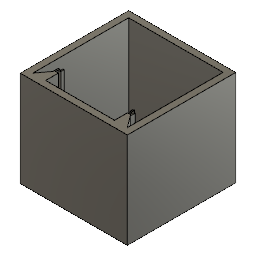
Albapod-V1 (Autodesk Fusion 360 design; units mm, degrees)
Autodesk Fusion 360 part; units mm, degrees
sketch "Sketch1" plane through (0, 0, 0) normal (0, 1, 0) x (1, 0, 0)
  line L0 (0, 0) -> (1, 0)
  line L1 (1, 0) -> (1, -1.5)
  line L2 (1, -1.5) -> (0, -1.5)
  line L3 (0, -1.5) -> (0, 0)
  line L4 (1, -1.5) -> (-2.25, -1.5)
  line L5 (-2.25, -1.5) -> (-2.25, -2.5)
  line L6 (-2.25, -2.5) -> (1, -2.5)
  line L7 (1, -2.5) -> (1, -1.5)
  line L8 (-2.25, -2.5) -> (-1.25, -2.5)
  line L9 (-1.25, -2.5) -> (-1.25, -4.5)
  line L10 (-1.25, -4.5) -> (-2.25, -4.5)
  line L11 (-2.25, -4.5) -> (-2.25, -2.5)
  line L12 (-2.25, -4.5) -> (1, -4.5)
  line L13 (1, -4.5) -> (1, -5.5)
  line L14 (1, -5.5) -> (-2.25, -5.5)
  line L15 (-2.25, -5.5) -> (-2.25, -4.5)
  line L16 (1, -5.5) -> (0, -5.5)
  line L17 (0, -5.5) -> (0, -14.5)
  line L18 (0, -14.5) -> (1, -14.5)
  line L19 (1, -14.5) -> (1, -5.5)
  line L20 (55, 0) -> (56, 0)
  line L21 (56, 0) -> (56, -1.5)
  line L22 (56, -1.5) -> (55, -1.5)
  line L23 (55, -1.5) -> (55, 0)
  line L24 (55, -1.5) -> (58.25, -1.5)
  line L25 (58.25, -1.5) -> (58.25, -2.5)
  line L26 (58.25, -2.5) -> (55, -2.5)
  line L27 (55, -2.5) -> (55, -1.5)
  line L28 (58.25, -2.5) -> (57.25, -2.5)
  line L29 (57.25, -2.5) -> (57.25, -4.5)
  line L30 (57.25, -4.5) -> (58.25, -4.5)
  line L31 (58.25, -4.5) -> (58.25, -2.5)
  line L32 (58.25, -4.5) -> (55, -4.5)
  line L33 (55, -4.5) -> (55, -5.5)
  line L34 (55, -5.5) -> (58.25, -5.5)
  line L35 (58.25, -5.5) -> (58.25, -4.5)
  line L36 (55, -5.5) -> (56, -5.5)
  line L37 (56, -5.5) -> (56, -14.5)
  line L38 (56, -14.5) -> (55, -14.5)
  line L39 (55, -14.5) -> (55, -5.5)
  line L40 (-9, -14.5) -> (65, -14.5)
  line L41 (65, -14.5) -> (65, 60.5)
  line L42 (65, 60.5) -> (-9, 60.5)
  line L43 (-9, 60.5) -> (-9, -14.5)
  line L44 (70, -19.5) -> (70, 65.5)
  line L45 (70, 65.5) -> (-14, 65.5)
  line L46 (-14, 65.5) -> (-14, -19.5)
  line L47 (-14, -19.5) -> (70, -19.5)
  line L48 (-2.25, -5.5) -> (-9, -14.5)
  line L49 (58.25, -5.5) -> (65, -14.5)
  dimension "d1" = 1
  dimension "d2" = 1.5
  dimension "d3" = 3.25
  dimension "d4" = 1
  dimension "d5" = 1
  dimension "d6" = 2
  dimension "d7" = 3.25
  dimension "d8" = 1
  dimension "d9" = 9
  dimension "d10" = 1.5
  dimension "d11" = 54
  dimension "d12" = 3.25
  dimension "d13" = 1
  dimension "d14" = 2
  dimension "d15" = 3.25
  dimension "d16" = 1
  dimension "d17" = 9
  dimension "d18" = 74
  dimension "d19" = 75
  dimension "d20" = 10
  dimension "d21" = 60.5
  dimension "d22" = 5
  constraint horizontal L0
  constraint vertical L1
  constraint horizontal L2
  constraint vertical L3
  constraint coincident L0.start L3.end
  constraint horizontal L4
  constraint vertical L5
  constraint horizontal L6
  constraint vertical L7
  constraint horizontal L8
  constraint vertical L9
  constraint horizontal L10
  constraint vertical L11
  constraint horizontal L12
  constraint vertical L13
  constraint horizontal L14
  constraint vertical L15
  constraint horizontal L16
  constraint vertical L17
  constraint horizontal L18
  constraint vertical L19
  constraint horizontal L20
  constraint vertical L21
  constraint horizontal L22
  constraint vertical L23
  constraint horizontal L24
  constraint vertical L25
  constraint horizontal L26
  constraint vertical L27
  constraint horizontal L28
  constraint vertical L29
  constraint horizontal L30
  constraint vertical L31
  constraint horizontal L32
  constraint vertical L33
  constraint horizontal L34
  constraint vertical L35
  constraint horizontal L36
  constraint vertical L37
  constraint horizontal L38
  constraint vertical L39
  constraint horizontal L40
  constraint vertical L41
  constraint horizontal L42
  constraint vertical L43
  measures "d1" distance of L0.start L0.end
  measures "d2" distance of L0.start L2.end
  measures "d3" distance of L1.end L4.end
  measures "d4" distance of L1.end L6.end
  measures "d5" distance of L5.end L8.end
  measures "d6" distance of L5.end L10.end
  measures "d7" distance of L10.end L12.end
  measures "d8" distance of L10.end L14.end
  measures "d9" distance of L13.end L18.end
  measures "d10" distance of L20.start L22.end
  measures "d11" distance of L1 L23
  measures "d12" distance of L22.end L24.end
  measures "d13" distance of L25.end L28.end
  measures "d14" distance of L25.end L30.end
  measures "d15" distance of L30.end L32.end
  measures "d16" distance of L30.end L34.end
  measures "d17" distance of L33.end L38.end
  measures "d18" distance of L40.start L40.end
  measures "d19" distance of L40.start L42.end
  measures "d20" distance of L19 L43
  measures "d21" distance of L0 L42
extrude "Extrude1" add sketch "Sketch1" along normal blind 75 contours L0 L1 L2 L3 L4 | L2 L4 L5 L6 L7 L8 | L6 L8 L9 L10 L11 L12 | L10 L12 L13 L14 L15 L16 | L14 L17 L40 L48 | L14 L16 L17 L18 L19 L40 | L34 L36 L37 L38 L39 L40 | L34 L37 L40 L49 | L30 L32 L33 L34 L35 L36 | L26 L28 L29 L30 L31 L32 | L22 L24 L25 L26 L27 L28 | L20 L21 L22 L23 L24 | L44 L45 L46 L47
equation "d20 = ( ( 74 - 54 ) / 2 ) * 1 mm"
